Autodesk Fusion 360 part; units mm, degrees
(part 5 of 9)
  spline S340 degree 3 poles (68.6306, 8.3911) (68.6068, 8.8872) (68.4218, 9.22) (68.0776, 9.3884) knots 0 0 0 0 1 1 1 1
  spline S341 degree 3 poles (68.0776, 9.3884) (67.8813, 9.4814) (67.5733, 9.528) (67.1526, 9.528) knots 0 0 0 0 1 1 1 1
  line L476 (67.1526, 9.528) -> (64.8117, 9.528)
  line L477 (64.8117, 9.528) -> (64.8117, 6.2723)
  line L478 (64.8117, 6.2723) -> (63.7833, 6.2723)
  line L479 (63.7833, 6.2723) -> (63.7833, 13.8636)
  line L480 (81.4443, 13.8636) -> (81.4443, 9.1714)
  spline S342 degree 3 poles (81.4443, 9.1714) (81.4443, 8.6205) (81.5476, 8.1616) (81.7543, 7.7968) knots 0 0 0 0 1 1 1 1
  spline S343 degree 3 poles (81.7543, 7.7968) (82.0613, 7.2459) (82.5781, 6.97) (83.3046, 6.97) knots 0 0 0 0 1 1 1 1
  spline S344 degree 3 poles (83.3046, 6.97) (84.1759, 6.97) (84.7691, 7.2676) (85.0823, 7.864) knots 0 0 0 0 1 1 1 1
  spline S345 degree 3 poles (85.0823, 7.864) (85.2508, 8.1875) (85.3355, 8.6236) (85.3355, 9.1714) knots 0 0 0 0 1 1 1 1
  line L481 (85.3355, 9.1714) -> (85.3355, 13.8636)
  line L482 (85.3355, 13.8636) -> (86.3794, 13.8636)
  line L483 (86.3794, 13.8636) -> (86.3794, 9.6003)
  spline S346 degree 3 poles (86.3794, 9.6003) (86.3794, 8.667) (86.2533, 7.9487) (86.0021, 7.4454) knots 0 0 0 0 1 1 1 1
  spline S347 degree 3 poles (86.0021, 7.4454) (85.5401, 6.5287) (84.6689, 6.0708) (83.3873, 6.0708) knots 0 0 0 0 1 1 1 1
  spline S348 degree 3 poles (83.3873, 6.0708) (82.1057, 6.0708) (81.2355, 6.5287) (80.7776, 7.4454) knots 0 0 0 0 1 1 1 1
  spline S349 degree 3 poles (80.7776, 7.4454) (80.5265, 7.9487) (80.4004, 8.667) (80.4004, 9.6003) knots 0 0 0 0 1 1 1 1
  line L484 (80.4004, 9.6003) -> (80.4004, 13.8636)
  line L485 (80.4004, 13.8636) -> (81.4443, 13.8636)
  line L486 (83.8782, 15.6619) -> (84.8446, 15.6619)
  line L487 (84.8446, 15.6619) -> (84.8446, 14.5871)
  line L488 (84.8446, 14.5871) -> (83.8782, 14.5871)
  line L489 (83.8782, 14.5871) -> (83.8782, 15.6619)
  line L490 (82.1729, 15.6619) -> (83.1393, 15.6619)
  line L491 (83.1393, 15.6619) -> (83.1393, 14.5871)
  line L492 (83.1393, 14.5871) -> (82.1729, 14.5871)
  line L493 (82.1729, 14.5871) -> (82.1729, 15.6619)
  line L494 (-85.4675, -4.6366) -> (-83.2868, -11.1013)
  line L495 (-83.2868, -11.1013) -> (-81.1319, -4.6366)
  line L496 (-81.1319, -4.6366) -> (-79.9795, -4.6366)
  line L497 (-79.9795, -4.6366) -> (-82.7493, -12.2278)
  line L498 (-82.7493, -12.2278) -> (-83.8397, -12.2278)
  line L499 (-83.8397, -12.2278) -> (-86.6044, -4.6366)
  line L500 (-86.6044, -4.6366) -> (-85.4675, -4.6366)
  line L501 (-67.1058, -4.6366) -> (-66.0671, -4.6366)
  line L502 (-66.0671, -4.6366) -> (-66.0671, -12.2278)
  line L503 (-66.0671, -12.2278) -> (-67.1058, -12.2278)
  line L504 (-67.1058, -12.2278) -> (-67.1058, -4.6366)
  line L505 (-52.6313, -4.6366) -> (-47.0967, -4.6366)
  line L506 (-47.0967, -4.6366) -> (-47.0967, -5.5667)
  line L507 (-47.0967, -5.5667) -> (-51.6287, -5.5667)
  line L508 (-51.6287, -5.5667) -> (-51.6287, -7.8715)
  line L509 (-51.6287, -7.8715) -> (-47.4378, -7.8715)
  line L510 (-47.4378, -7.8715) -> (-47.4378, -8.75)
  line L511 (-47.4378, -8.75) -> (-51.6287, -8.75)
  line L512 (-51.6287, -8.75) -> (-51.6287, -11.3235)
  line L513 (-51.6287, -11.3235) -> (-47.0192, -11.3235)
  line L514 (-47.0192, -11.3235) -> (-47.0192, -12.2278)
  line L515 (-47.0192, -12.2278) -> (-52.6313, -12.2278)
  line L516 (-52.6313, -12.2278) -> (-52.6313, -4.6366)
  spline S350 degree 3 poles (-32.8237, -8.1144) (-32.341, -8.1144) (-31.9597, -8.0183) (-31.6796, -7.825) knots 0 0 0 0 1 1 1 1
  spline S351 degree 3 poles (-31.6796, -7.825) (-31.3985, -7.6317) (-31.2579, -7.2845) (-31.2579, -6.7811) knots 0 0 0 0 1 1 1 1
  spline S352 degree 3 poles (-31.2579, -6.7811) (-31.2579, -6.2406) (-31.4543, -5.8716) (-31.847, -5.6753) knots 0 0 0 0 1 1 1 1
  spline S353 degree 3 poles (-31.847, -5.6753) (-32.0568, -5.5719) (-32.3379, -5.5202) (-32.6893, -5.5202) knots 0 0 0 0 1 1 1 1
  line L517 (-32.6893, -5.5202) -> (-35.2008, -5.5202)
  line L518 (-35.2008, -5.5202) -> (-35.2008, -8.1144)
  line L519 (-35.2008, -8.1144) -> (-32.8237, -8.1144)
  line L520 (-36.2292, -4.6366) -> (-32.7152, -4.6366)
  spline S354 degree 3 poles (-32.7152, -4.6366) (-32.1364, -4.6366) (-31.6589, -4.7213) (-31.2837, -4.8898) knots 0 0 0 0 1 1 1 1
  spline S355 degree 3 poles (-31.2837, -4.8898) (-30.5706, -5.2133) (-30.214, -5.8117) (-30.214, -6.6829) knots 0 0 0 0 1 1 1 1
  spline S356 degree 3 poles (-30.214, -6.6829) (-30.214, -7.1377) (-30.3081, -7.5098) (-30.4951, -7.7992) knots 0 0 0 0 1 1 1 1
  spline S357 degree 3 poles (-30.4951, -7.7992) (-30.6833, -8.0885) (-30.9458, -8.3211) (-31.2837, -8.4968) knots 0 0 0 0 1 1 1 1
  spline S358 degree 3 poles (-31.2837, -8.4968) (-30.9871, -8.6177) (-30.7639, -8.7758) (-30.615, -8.9722) knots 0 0 0 0 1 1 1 1
  spline S359 degree 3 poles (-30.615, -8.9722) (-30.4652, -9.1686) (-30.3815, -9.4869) (-30.3639, -9.9282) knots 0 0 0 0 1 1 1 1
  line L521 (-30.3639, -9.9282) -> (-30.3277, -10.9462)
  spline S360 degree 3 poles (-30.3277, -10.9462) (-30.3174, -11.2356) (-30.2936, -11.4506) (-30.2554, -11.5922) knots 0 0 0 0 1 1 1 1
  spline S361 degree 3 poles (-30.2554, -11.5922) (-30.1934, -11.833) (-30.0828, -11.988) (-29.9246, -12.0573) knots 0 0 0 0 1 1 1 1
  line L522 (-29.9246, -12.0573) -> (-29.9246, -12.2278)
  line L523 (-29.9246, -12.2278) -> (-31.1855, -12.2278)
  spline S362 degree 3 poles (-31.1855, -12.2278) (-31.2197, -12.1627) (-31.2476, -12.078) (-31.2682, -11.9746) knots 0 0 0 0 1 1 1 1
  spline S363 degree 3 poles (-31.2682, -11.9746) (-31.2889, -11.8713) (-31.3065, -11.6718) (-31.3199, -11.3752) knots 0 0 0 0 1 1 1 1
  line L524 (-31.3199, -11.3752) -> (-31.3819, -10.1091)
  spline S364 degree 3 poles (-31.3819, -10.1091) (-31.4057, -9.613) (-31.5907, -9.2802) (-31.9349, -9.1117) knots 0 0 0 0 1 1 1 1
  spline S365 degree 3 poles (-31.9349, -9.1117) (-32.1312, -9.0187) (-32.4392, -8.9722) (-32.8599, -8.9722) knots 0 0 0 0 1 1 1 1
  line L525 (-32.8599, -8.9722) -> (-35.2008, -8.9722)
  line L526 (-35.2008, -8.9722) -> (-35.2008, -12.2278)
  line L527 (-35.2008, -12.2278) -> (-36.2292, -12.2278)
  line L528 (-36.2292, -12.2278) -> (-36.2292, -4.6366)
  line L529 (-17.0996, -4.6366) -> (-16.0609, -4.6366)
  line L530 (-16.0609, -4.6366) -> (-16.0609, -12.2278)
  line L531 (-16.0609, -12.2278) -> (-17.0996, -12.2278)
  line L532 (-17.0996, -12.2278) -> (-17.0996, -4.6366)
  line L533 (-2.3284, -4.6366) -> (2.9374, -4.6366)
  line L534 (2.9374, -4.6366) -> (2.9374, -5.5667)
  line L535 (2.9374, -5.5667) -> (-1.3, -5.5667)
  line L536 (-1.3, -5.5667) -> (-1.3, -7.8715)
  line L537 (-1.3, -7.8715) -> (2.4258, -7.8715)
  line L538 (2.4258, -7.8715) -> (2.4258, -8.7758)
  line L539 (2.4258, -8.7758) -> (-1.3, -8.7758)
  line L540 (-1.3, -8.7758) -> (-1.3, -12.2278)
  line L541 (-1.3, -12.2278) -> (-2.3284, -12.2278)
  line L542 (-2.3284, -12.2278) -> (-2.3284, -4.6366)
  line L543 (14.7693, -4.6366) -> (14.7693, -9.3288)
  spline S366 degree 3 poles (14.7693, -9.3288) (14.7693, -9.8796) (14.8726, -10.3385) (15.0793, -10.7034) knots 0 0 0 0 1 1 1 1
  spline S367 degree 3 poles (15.0793, -10.7034) (15.3863, -11.2542) (15.9031, -11.5302) (16.6296, -11.5302) knots 0 0 0 0 1 1 1 1
  spline S368 degree 3 poles (16.6296, -11.5302) (17.5009, -11.5302) (18.0941, -11.2325) (18.4073, -10.6362) knots 0 0 0 0 1 1 1 1
  spline S369 degree 3 poles (18.4073, -10.6362) (18.5758, -10.3127) (18.6605, -9.8765) (18.6605, -9.3288) knots 0 0 0 0 1 1 1 1
  line L544 (18.6605, -9.3288) -> (18.6605, -4.6366)
  line L545 (18.6605, -4.6366) -> (19.7044, -4.6366)
  line L546 (19.7044, -4.6366) -> (19.7044, -8.8999)
  spline S370 degree 3 poles (19.7044, -8.8999) (19.7044, -9.8331) (19.5783, -10.5514) (19.3271, -11.0548) knots 0 0 0 0 1 1 1 1
  spline S371 degree 3 poles (19.3271, -11.0548) (18.8651, -11.9715) (17.9939, -12.4294) (16.7123, -12.4294) knots 0 0 0 0 1 1 1 1
  spline S372 degree 3 poles (16.7123, -12.4294) (15.4307, -12.4294) (14.5605, -11.9715) (14.1026, -11.0548) knots 0 0 0 0 1 1 1 1
  spline S373 degree 3 poles (14.1026, -11.0548) (13.8515, -10.5514) (13.7254, -9.8331) (13.7254, -8.8999) knots 0 0 0 0 1 1 1 1
  line L547 (13.7254, -8.8999) -> (13.7254, -4.6366)
  line L548 (13.7254, -4.6366) -> (14.7693, -4.6366)
  line L549 (17.2032, -2.8382) -> (18.1696, -2.8382)
  line L550 (18.1696, -2.8382) -> (18.1696, -3.9131)
  line L551 (18.1696, -3.9131) -> (17.2032, -3.9131)
  line L552 (17.2032, -3.9131) -> (17.2032, -2.8382)
  line L553 (15.4979, -2.8382) -> (16.4643, -2.8382)
  line L554 (16.4643, -2.8382) -> (16.4643, -3.9131)
  line L555 (16.4643, -3.9131) -> (15.4979, -3.9131)
  line L556 (15.4979, -3.9131) -> (15.4979, -2.8382)
  line L557 (31.0091, -4.6366) -> (36.2749, -4.6366)
  line L558 (36.2749, -4.6366) -> (36.2749, -5.5667)
  line L559 (36.2749, -5.5667) -> (32.0375, -5.5667)
  line L560 (32.0375, -5.5667) -> (32.0375, -7.8715)
  line L561 (32.0375, -7.8715) -> (35.7633, -7.8715)
  line L562 (35.7633, -7.8715) -> (35.7633, -8.7758)
  line L563 (35.7633, -8.7758) -> (32.0375, -8.7758)
  line L564 (32.0375, -8.7758) -> (32.0375, -12.2278)
  line L565 (32.0375, -12.2278) -> (31.0091, -12.2278)
  line L566 (31.0091, -12.2278) -> (31.0091, -4.6366)
  line L567 (49.5754, -4.6366) -> (50.6141, -4.6366)
  line L568 (50.6141, -4.6366) -> (50.6141, -12.2278)
  line L569 (50.6141, -12.2278) -> (49.5754, -12.2278)
  line L570 (49.5754, -12.2278) -> (49.5754, -4.6366)
  spline S374 degree 3 poles (64.6236, -9.7784) (64.6474, -10.2093) (64.7497, -10.5587) (64.9285, -10.8274) knots 0 0 0 0 1 1 1 1
  spline S375 degree 3 poles (64.9285, -10.8274) (65.2695, -11.3307) (65.8711, -11.5819) (66.732, -11.5819) knots 0 0 0 0 1 1 1 1
  spline S376 degree 3 poles (66.732, -11.5819) (67.1175, -11.5819) (67.4689, -11.5271) (67.7862, -11.4165) knots 0 0 0 0 1 1 1 1
  spline S377 degree 3 poles (67.7862, -11.4165) (68.3991, -11.2026) (68.706, -10.8202) (68.706, -10.2693) knots 0 0 0 0 1 1 1 1
  spline S378 degree 3 poles (68.706, -10.2693) (68.706, -9.8559) (68.5768, -9.5613) (68.3185, -9.3856) knots 0 0 0 0 1 1 1 1
  spline S379 degree 3 poles (68.3185, -9.3856) (68.057, -9.213) (67.6467, -9.0632) (67.0886, -8.936) knots 0 0 0 0 1 1 1 1
  line L571 (67.0886, -8.936) -> (66.0602, -8.7035)
  spline S380 degree 3 poles (66.0602, -8.7035) (65.3884, -8.5516) (64.913, -8.3852) (64.6339, -8.2022) knots 0 0 0 0 1 1 1 1
  spline S381 degree 3 poles (64.6339, -8.2022) (64.1513, -7.8849) (63.9105, -7.4116) (63.9105, -6.7811) knots 0 0 0 0 1 1 1 1
  spline S382 degree 3 poles (63.9105, -6.7811) (63.9105, -6.099) (64.1461, -5.5388) (64.6184, -5.1016) knots 0 0 0 0 1 1 1 1
  spline S383 degree 3 poles (64.6184, -5.1016) (65.0907, -4.6645) (65.7584, -4.4454) (66.6235, -4.4454) knots 0 0 0 0 1 1 1 1
  spline S384 degree 3 poles (66.6235, -4.4454) (67.4193, -4.4454) (68.0952, -4.6376) (68.6523, -5.0221) knots 0 0 0 0 1 1 1 1
  spline S385 degree 3 poles (68.6523, -5.0221) (69.2083, -5.4055) (69.4863, -6.0194) (69.4863, -6.8638) knots 0 0 0 0 1 1 1 1
  line L572 (69.4863, -6.8638) -> (68.52, -6.8638)
  spline S386 degree 3 poles (68.52, -6.8638) (68.4683, -6.4576) (68.3577, -6.1455) (68.1893, -5.9285) knots 0 0 0 0 1 1 1 1
  spline S387 degree 3 poles (68.1893, -5.9285) (67.8761, -5.5326) (67.3438, -5.3342) (66.5925, -5.3342) knots 0 0 0 0 1 1 1 1
  spline S388 degree 3 poles (66.5925, -5.3342) (65.9858, -5.3342) (65.5507, -5.4613) (65.2851, -5.7166) knots 0 0 0 0 1 1 1 1
  spline S389 degree 3 poles (65.2851, -5.7166) (65.0194, -5.9719) (64.8871, -6.2675) (64.8871, -6.6054) knots 0 0 0 0 1 1 1 1
  spline S390 degree 3 poles (64.8871, -6.6054) (64.8871, -6.9775) (65.0422, -7.2493) (65.3522, -7.4219) knots 0 0 0 0 1 1 1 1
  spline S391 degree 3 poles (65.3522, -7.4219) (65.5558, -7.5325) (66.0158, -7.67) (66.732, -7.8353) knots 0 0 0 0 1 1 1 1
  line L573 (66.732, -7.8353) -> (67.7965, -8.0782)
  spline S392 degree 3 poles (67.7965, -8.0782) (68.3102, -8.195) (68.706, -8.3552) (68.9851, -8.5588) knots 0 0 0 0 1 1 1 1
  spline S393 degree 3 poles (68.9851, -8.5588) (69.4677, -8.9133) (69.7086, -9.429) (69.7086, -10.1039) knots 0 0 0 0 1 1 1 1
  spline S394 degree 3 poles (69.7086, -10.1039) (69.7086, -10.9442) (69.4026, -11.5457) (68.7908, -11.9074) knots 0 0 0 0 1 1 1 1
  spline S395 degree 3 poles (68.7908, -11.9074) (68.18, -12.2692) (67.4689, -12.45) (66.6596, -12.45) knots 0 0 0 0 1 1 1 1
  spline S396 degree 3 poles (66.6596, -12.45) (65.716, -12.45) (64.9771, -12.2092) (64.4427, -11.7266) knots 0 0 0 0 1 1 1 1
  spline S397 degree 3 poles (64.4427, -11.7266) (63.9084, -11.248) (63.6469, -10.5979) (63.6572, -9.7784) knots 0 0 0 0 1 1 1 1
  line L574 (63.6572, -9.7784) -> (64.6236, -9.7784)
  line L575 (86.4414, -4.6366) -> (86.4414, -5.5409)
  line L576 (86.4414, -5.5409) -> (83.8834, -5.5409)
  line L577 (83.8834, -5.5409) -> (83.8834, -12.2278)
  line L578 (83.8834, -12.2278) -> (82.8395, -12.2278)
  line L579 (82.8395, -12.2278) -> (82.8395, -5.5409)
  line L580 (82.8395, -5.5409) -> (80.2816, -5.5409)
  line L581 (80.2816, -5.5409) -> (80.2816, -4.6366)
  line L582 (80.2816, -4.6366) -> (86.4414, -4.6366)
  spline S398 degree 3 poles (-85.3952, -28.2785) (-85.3714, -28.7095) (-85.2691, -29.0588) (-85.0903, -29.3276) knots 0 0 0 0 1 1 1 1
  spline S399 degree 3 poles (-85.0903, -29.3276) (-84.7492, -29.8309) (-84.1477, -30.082) (-83.2868, -30.082) knots 0 0 0 0 1 1 1 1
  spline S400 degree 3 poles (-83.2868, -30.082) (-82.9013, -30.082) (-82.5499, -30.0273) (-82.2326, -29.9167) knots 0 0 0 0 1 1 1 1
  spline S401 degree 3 poles (-82.2326, -29.9167) (-81.6197, -29.7027) (-81.3127, -29.3203) (-81.3127, -28.7694) knots 0 0 0 0 1 1 1 1
  spline S402 degree 3 poles (-81.3127, -28.7694) (-81.3127, -28.356) (-81.4419, -28.0615) (-81.7003, -27.8858) knots 0 0 0 0 1 1 1 1
  spline S403 degree 3 poles (-81.7003, -27.8858) (-81.9618, -27.7132) (-82.3721, -27.5633) (-82.9302, -27.4362) knots 0 0 0 0 1 1 1 1
  line L583 (-82.9302, -27.4362) -> (-83.9586, -27.2037)
  spline S404 degree 3 poles (-83.9586, -27.2037) (-84.6303, -27.0517) (-85.1058, -26.8853) (-85.3848, -26.7024) knots 0 0 0 0 1 1 1 1
  spline S405 degree 3 poles (-85.3848, -26.7024) (-85.8675, -26.3851) (-86.1083, -25.9117) (-86.1083, -25.2813) knots 0 0 0 0 1 1 1 1
  spline S406 degree 3 poles (-86.1083, -25.2813) (-86.1083, -24.5992) (-85.8726, -24.039) (-85.4003, -23.6018) knots 0 0 0 0 1 1 1 1
  spline S407 degree 3 poles (-85.4003, -23.6018) (-84.928, -23.1646) (-84.2603, -22.9455) (-83.3953, -22.9455) knots 0 0 0 0 1 1 1 1
  spline S408 degree 3 poles (-83.3953, -22.9455) (-82.5995, -22.9455) (-81.9235, -23.1378) (-81.3665, -23.5222) knots 0 0 0 0 1 1 1 1
  spline S409 degree 3 poles (-81.3665, -23.5222) (-80.8104, -23.9057) (-80.5324, -24.5196) (-80.5324, -25.364) knots 0 0 0 0 1 1 1 1
  line L584 (-80.5324, -25.364) -> (-81.4988, -25.364)
  spline S410 degree 3 poles (-81.4988, -25.364) (-81.5504, -24.9578) (-81.661, -24.6457) (-81.8295, -24.4286) knots 0 0 0 0 1 1 1 1
  spline S411 degree 3 poles (-81.8295, -24.4286) (-82.1426, -24.0328) (-82.6749, -23.8344) (-83.4263, -23.8344) knots 0 0 0 0 1 1 1 1
  spline S412 degree 3 poles (-83.4263, -23.8344) (-84.033, -23.8344) (-84.4681, -23.9615) (-84.7337, -24.2168) knots 0 0 0 0 1 1 1 1
  spline S413 degree 3 poles (-84.7337, -24.2168) (-84.9993, -24.472) (-85.1316, -24.7676) (-85.1316, -25.1056) knots 0 0 0 0 1 1 1 1
  spline S414 degree 3 poles (-85.1316, -25.1056) (-85.1316, -25.4777) (-84.9766, -25.7495) (-84.6665, -25.9221) knots 0 0 0 0 1 1 1 1
  spline S415 degree 3 poles (-84.6665, -25.9221) (-84.4629, -26.0327) (-84.003, -26.1701) (-83.2868, -26.3355) knots 0 0 0 0 1 1 1 1
  line L585 (-83.2868, -26.3355) -> (-82.2222, -26.5784)
  spline S416 degree 3 poles (-82.2222, -26.5784) (-81.7086, -26.6952) (-81.3127, -26.8554) (-81.0337, -27.059) knots 0 0 0 0 1 1 1 1
  spline S417 degree 3 poles (-81.0337, -27.059) (-80.551, -27.4135) (-80.3102, -27.9292) (-80.3102, -28.6041) knots 0 0 0 0 1 1 1 1
  spline S418 degree 3 poles (-80.3102, -28.6041) (-80.3102, -29.4443) (-80.6161, -30.0459) (-81.228, -30.4076) knots 0 0 0 0 1 1 1 1
  spline S419 degree 3 poles (-81.228, -30.4076) (-81.8388, -30.7693) (-82.5499, -30.9502) (-83.3591, -30.9502) knots 0 0 0 0 1 1 1 1
  spline S420 degree 3 poles (-83.3591, -30.9502) (-84.3027, -30.9502) (-85.0417, -30.7094) (-85.576, -30.2267) knots 0 0 0 0 1 1 1 1
  spline S421 degree 3 poles (-85.576, -30.2267) (-86.1104, -29.7482) (-86.3718, -29.0981) (-86.3615, -28.2785) knots 0 0 0 0 1 1 1 1
  line L586 (-86.3615, -28.2785) -> (-85.3952, -28.2785)
  line L587 (-65.5018, -27.6171) -> (-66.6542, -24.2633)
  line L588 (-66.6542, -24.2633) -> (-67.8789, -27.6171)
  line L589 (-67.8789, -27.6171) -> (-65.5018, -27.6171)
  line L590 (-67.1916, -23.1367) -> (-66.0289, -23.1367)
  line L591 (-66.0289, -23.1367) -> (-63.2745, -30.728)
  line L592 (-63.2745, -30.728) -> (-64.4011, -30.728)
  line L593 (-64.4011, -30.728) -> (-65.1711, -28.4542)
  line L594 (-65.1711, -28.4542) -> (-68.1735, -28.4542)
  line L595 (-68.1735, -28.4542) -> (-68.9951, -30.728)
  line L596 (-68.9951, -30.728) -> (-70.0493, -30.728)
  line L597 (-70.0493, -30.728) -> (-67.1916, -23.1367)
  line L598 (-66.2924, -21.3384) -> (-65.3261, -21.3384)
  line L599 (-65.3261, -21.3384) -> (-65.3261, -22.4132)
  line L600 (-65.3261, -22.4132) -> (-66.2924, -22.4132)
  line L601 (-66.2924, -22.4132) -> (-66.2924, -21.3384)
  line L602 (-67.9978, -21.3384) -> (-67.0314, -21.3384)
  line L603 (-67.0314, -21.3384) -> (-67.0314, -22.4132)
  line L604 (-67.0314, -22.4132) -> (-67.9978, -22.4132)
  line L605 (-67.9978, -22.4132) -> (-67.9978, -21.3384)
  spline S422 degree 3 poles (-49.8232, -22.93) (-48.862, -22.93) (-48.1158, -23.1832) (-47.5856, -23.6897) knots 0 0 0 0 1 1 1 1
  spline S423 degree 3 poles (-47.5856, -23.6897) (-47.0554, -24.1961) (-46.7608, -24.7718) (-46.7019, -25.4156) knots 0 0 0 0 1 1 1 1
  line L606 (-46.7019, -25.4156) -> (-47.7044, -25.4156)
  spline S424 degree 3 poles (-47.7044, -25.4156) (-47.8181, -24.9268) (-48.0445, -24.5392) (-48.3835, -24.2529) knots 0 0 0 0 1 1 1 1
  spline S425 degree 3 poles (-48.3835, -24.2529) (-48.7235, -23.9666) (-49.2, -23.824) (-49.8128, -23.824) knots 0 0 0 0 1 1 1 1
  spline S426 degree 3 poles (-49.8128, -23.824) (-50.5601, -23.824) (-51.1637, -24.0865) (-51.6246, -24.6116) knots 0 0 0 0 1 1 1 1
  spline S427 degree 3 poles (-51.6246, -24.6116) (-52.0845, -25.1376) (-52.314, -25.9427) (-52.314, -27.028) knots 0 0 0 0 1 1 1 1
  spline S428 degree 3 poles (-52.314, -27.028) (-52.314, -27.9168) (-52.1062, -28.6382) (-51.6908, -29.1901) knots 0 0 0 0 1 1 1 1
  spline S429 degree 3 poles (-51.6908, -29.1901) (-51.2763, -29.743) (-50.6572, -30.02) (-49.8335, -30.02) knots 0 0 0 0 1 1 1 1
  spline S430 degree 3 poles (-49.8335, -30.02) (-49.0759, -30.02) (-48.4982, -29.7286) (-48.1023, -29.1467) knots 0 0 0 0 1 1 1 1
  spline S431 degree 3 poles (-48.1023, -29.1467) (-47.8925, -28.8397) (-47.7354, -28.4367) (-47.6321, -27.9375) knots 0 0 0 0 1 1 1 1
  line L607 (-47.6321, -27.9375) -> (-46.6296, -27.9375)
  spline S432 degree 3 poles (-46.6296, -27.9375) (-46.7195, -28.7364) (-47.0151, -29.4071) (-47.5184, -29.9477) knots 0 0 0 0 1 1 1 1
  spline S433 degree 3 poles (-47.5184, -29.9477) (-48.1209, -30.5988) (-48.9343, -30.9244) (-49.9575, -30.9244) knots 0 0 0 0 1 1 1 1
  spline S434 degree 3 poles (-49.9575, -30.9244) (-50.8391, -30.9244) (-51.5802, -30.6577) (-52.1796, -30.1234) knots 0 0 0 0 1 1 1 1
  spline S435 degree 3 poles (-52.1796, -30.1234) (-52.9682, -29.4175) (-53.363, -28.3271) (-53.363, -26.8523) knots 0 0 0 0 1 1 1 1
  spline S436 degree 3 poles (-53.363, -26.8523) (-53.363, -25.7329) (-53.0664, -24.8141) (-52.4742, -24.0979) knots 0 0 0 0 1 1 1 1
  spline S437 degree 3 poles (-52.4742, -24.0979) (-51.8334, -23.3197) (-50.9497, -22.93) (-49.8232, -22.93) knots 0 0 0 0 1 1 1 1
  line L608 (-36.3274, -23.1367) -> (-35.2887, -23.1367)
  line L609 (-35.2887, -23.1367) -> (-35.2887, -26.2735)
  line L610 (-35.2887, -26.2735) -> (-31.3406, -26.2735)
  line L611 (-31.3406, -26.2735) -> (-31.3406, -23.1367)
  line L612 (-31.3406, -23.1367) -> (-30.3019, -23.1367)
  line L613 (-30.3019, -23.1367) -> (-30.3019, -30.728)
  line L614 (-30.3019, -30.728) -> (-31.3406, -30.728)
  line L615 (-31.3406, -30.728) -> (-31.3406, -27.1778)
  line L616 (-31.3406, -27.1778) -> (-35.2887, -27.1778)
  line L617 (-35.2887, -27.1778) -> (-35.2887, -30.728)
  line L618 (-35.2887, -30.728) -> (-36.3274, -30.728)
  line L619 (-36.3274, -30.728) -> (-36.3274, -23.1367)
  spline S438 degree 3 poles (-18.7202, -28.2785) (-18.6964, -28.7095) (-18.5941, -29.0588) (-18.4153, -29.3276) knots 0 0 0 0 1 1 1 1
  spline S439 degree 3 poles (-18.4153, -29.3276) (-18.0742, -29.8309) (-17.4727, -30.082) (-16.6118, -30.082) knots 0 0 0 0 1 1 1 1
  spline S440 degree 3 poles (-16.6118, -30.082) (-16.2263, -30.082) (-15.8749, -30.0273) (-15.5576, -29.9167) knots 0 0 0 0 1 1 1 1
  spline S441 degree 3 poles (-15.5576, -29.9167) (-14.9447, -29.7027) (-14.6377, -29.3203) (-14.6377, -28.7694) knots 0 0 0 0 1 1 1 1
  spline S442 degree 3 poles (-14.6377, -28.7694) (-14.6377, -28.356) (-14.7669, -28.0615) (-15.0253, -27.8858) knots 0 0 0 0 1 1 1 1
  spline S443 degree 3 poles (-15.0253, -27.8858) (-15.2868, -27.7132) (-15.6971, -27.5633) (-16.2552, -27.4362) knots 0 0 0 0 1 1 1 1
  line L620 (-16.2552, -27.4362) -> (-17.2836, -27.2037)
  spline S444 degree 3 poles (-17.2836, -27.2037) (-17.9553, -27.0517) (-18.4308, -26.8853) (-18.7098, -26.7024) knots 0 0 0 0 1 1 1 1
  spline S445 degree 3 poles (-18.7098, -26.7024) (-19.1925, -26.3851) (-19.4333, -25.9117) (-19.4333, -25.2813) knots 0 0 0 0 1 1 1 1
  spline S446 degree 3 poles (-19.4333, -25.2813) (-19.4333, -24.5992) (-19.1976, -24.039) (-18.7253, -23.6018) knots 0 0 0 0 1 1 1 1
  spline S447 degree 3 poles (-18.7253, -23.6018) (-18.253, -23.1646) (-17.5853, -22.9455) (-16.7203, -22.9455) knots 0 0 0 0 1 1 1 1
  spline S448 degree 3 poles (-16.7203, -22.9455) (-15.9245, -22.9455) (-15.2485, -23.1378) (-14.6915, -23.5222) knots 0 0 0 0 1 1 1 1
  spline S449 degree 3 poles (-14.6915, -23.5222) (-14.1354, -23.9057) (-13.8574, -24.5196) (-13.8574, -25.364) knots 0 0 0 0 1 1 1 1
  line L621 (-13.8574, -25.364) -> (-14.8238, -25.364)
  spline S450 degree 3 poles (-14.8238, -25.364) (-14.8754, -24.9578) (-14.986, -24.6457) (-15.1545, -24.4286) knots 0 0 0 0 1 1 1 1
  spline S451 degree 3 poles (-15.1545, -24.4286) (-15.4676, -24.0328) (-15.9999, -23.8344) (-16.7513, -23.8344) knots 0 0 0 0 1 1 1 1
  spline S452 degree 3 poles (-16.7513, -23.8344) (-17.358, -23.8344) (-17.7931, -23.9615) (-18.0587, -24.2168) knots 0 0 0 0 1 1 1 1
  spline S453 degree 3 poles (-18.0587, -24.2168) (-18.3243, -24.472) (-18.4566, -24.7676) (-18.4566, -25.1056) knots 0 0 0 0 1 1 1 1
  spline S454 degree 3 poles (-18.4566, -25.1056) (-18.4566, -25.4777) (-18.3016, -25.7495) (-17.9915, -25.9221) knots 0 0 0 0 1 1 1 1
  spline S455 degree 3 poles (-17.9915, -25.9221) (-17.7879, -26.0327) (-17.328, -26.1701) (-16.6118, -26.3355) knots 0 0 0 0 1 1 1 1
  line L622 (-16.6118, -26.3355) -> (-15.5472, -26.5784)
  spline S456 degree 3 poles (-15.5472, -26.5784) (-15.0336, -26.6952) (-14.6377, -26.8554) (-14.3587, -27.059) knots 0 0 0 0 1 1 1 1
  spline S457 degree 3 poles (-14.3587, -27.059) (-13.876, -27.4135) (-13.6352, -27.9292) (-13.6352, -28.6041) knots 0 0 0 0 1 1 1 1
  spline S458 degree 3 poles (-13.6352, -28.6041) (-13.6352, -29.4443) (-13.9411, -30.0459) (-14.553, -30.4076) knots 0 0 0 0 1 1 1 1
  spline S459 degree 3 poles (-14.553, -30.4076) (-15.1638, -30.7693) (-15.8749, -30.9502) (-16.6841, -30.9502) knots 0 0 0 0 1 1 1 1
  spline S460 degree 3 poles (-16.6841, -30.9502) (-17.6277, -30.9502) (-18.3667, -30.7094) (-18.901, -30.2267) knots 0 0 0 0 1 1 1 1
  spline S461 degree 3 poles (-18.901, -30.2267) (-19.4354, -29.7482) (-19.6968, -29.0981) (-19.6865, -28.2785) knots 0 0 0 0 1 1 1 1
  line L623 (-19.6865, -28.2785) -> (-18.7202, -28.2785)
  line L624 (-0.4308, -23.1367) -> (0.6079, -23.1367)
  line L625 (0.6079, -23.1367) -> (0.6079, -30.728)
  line L626 (0.6079, -30.728) -> (-0.4308, -30.728)
  line L627 (-0.4308, -30.728) -> (-0.4308, -23.1367)
  spline S462 degree 3 poles (14.6173, -28.2785) (14.6411, -28.7095) (14.7434, -29.0588) (14.9222, -29.3276) knots 0 0 0 0 1 1 1 1
  spline S463 degree 3 poles (14.9222, -29.3276) (15.2633, -29.8309) (15.8648, -30.082) (16.7257, -30.082) knots 0 0 0 0 1 1 1 1
  spline S464 degree 3 poles (16.7257, -30.082) (17.1112, -30.082) (17.4626, -30.0273) (17.7799, -29.9167) knots 0 0 0 0 1 1 1 1
  spline S465 degree 3 poles (17.7799, -29.9167) (18.3928, -29.7027) (18.6998, -29.3203) (18.6998, -28.7694) knots 0 0 0 0 1 1 1 1
  spline S466 degree 3 poles (18.6998, -28.7694) (18.6998, -28.356) (18.5706, -28.0615) (18.3122, -27.8858) knots 0 0 0 0 1 1 1 1
  spline S467 degree 3 poles (18.3122, -27.8858) (18.0507, -27.7132) (17.6404, -27.5633) (17.0823, -27.4362) knots 0 0 0 0 1 1 1 1
  line L628 (17.0823, -27.4362) -> (16.0539, -27.2037)
  spline S468 degree 3 poles (16.0539, -27.2037) (15.3822, -27.0517) (14.9067, -26.8853) (14.6277, -26.7024) knots 0 0 0 0 1 1 1 1
  spline S469 degree 3 poles (14.6277, -26.7024) (14.145, -26.3851) (13.9042, -25.9117) (13.9042, -25.2813) knots 0 0 0 0 1 1 1 1
  spline S470 degree 3 poles (13.9042, -25.2813) (13.9042, -24.5992) (14.1399, -24.039) (14.6122, -23.6018) knots 0 0 0 0 1 1 1 1
  spline S471 degree 3 poles (14.6122, -23.6018) (15.0845, -23.1646) (15.7522, -22.9455) (16.6172, -22.9455) knots 0 0 0 0 1 1 1 1
  spline S472 degree 3 poles (16.6172, -22.9455) (17.413, -22.9455) (18.089, -23.1378) (18.646, -23.5222) knots 0 0 0 0 1 1 1 1
  spline S473 degree 3 poles (18.646, -23.5222) (19.2021, -23.9057) (19.4801, -24.5196) (19.4801, -25.364) knots 0 0 0 0 1 1 1 1
  line L629 (19.4801, -25.364) -> (18.5137, -25.364)
  spline S474 degree 3 poles (18.5137, -25.364) (18.4621, -24.9578) (18.3515, -24.6457) (18.183, -24.4286) knots 0 0 0 0 1 1 1 1
  spline S475 degree 3 poles (18.183, -24.4286) (17.8699, -24.0328) (17.3376, -23.8344) (16.5862, -23.8344) knots 0 0 0 0 1 1 1 1
  spline S476 degree 3 poles (16.5862, -23.8344) (15.9795, -23.8344) (15.5444, -23.9615) (15.2788, -24.2168) knots 0 0 0 0 1 1 1 1
  spline S477 degree 3 poles (15.2788, -24.2168) (15.0132, -24.472) (14.8809, -24.7676) (14.8809, -25.1056) knots 0 0 0 0 1 1 1 1
  spline S478 degree 3 poles (14.8809, -25.1056) (14.8809, -25.4777) (15.0359, -25.7495) (15.346, -25.9221) knots 0 0 0 0 1 1 1 1
  spline S479 degree 3 poles (15.346, -25.9221) (15.5496, -26.0327) (16.0095, -26.1701) (16.7257, -26.3355) knots 0 0 0 0 1 1 1 1
  line L630 (16.7257, -26.3355) -> (17.7903, -26.5784)
  spline S480 degree 3 poles (17.7903, -26.5784) (18.3039, -26.6952) (18.6998, -26.8554) (18.9788, -27.059) knots 0 0 0 0 1 1 1 1
  spline S481 degree 3 poles (18.9788, -27.059) (19.4615, -27.4135) (19.7023, -27.9292) (19.7023, -28.6041) knots 0 0 0 0 1 1 1 1
  spline S482 degree 3 poles (19.7023, -28.6041) (19.7023, -29.4443) (19.3964, -30.0459) (18.7845, -30.4076) knots 0 0 0 0 1 1 1 1
  spline S483 degree 3 poles (18.7845, -30.4076) (18.1737, -30.7693) (17.4626, -30.9502) (16.6534, -30.9502) knots 0 0 0 0 1 1 1 1
  spline S484 degree 3 poles (16.6534, -30.9502) (15.7098, -30.9502) (14.9708, -30.7094) (14.4365, -30.2267) knots 0 0 0 0 1 1 1 1
  spline S485 degree 3 poles (14.4365, -30.2267) (13.9021, -29.7482) (13.6407, -29.0981) (13.651, -28.2785) knots 0 0 0 0 1 1 1 1
  line L631 (13.651, -28.2785) -> (14.6173, -28.2785)
  line L632 (32.9067, -23.1367) -> (33.9454, -23.1367)
  line L633 (33.9454, -23.1367) -> (33.9454, -30.728)
  line L634 (33.9454, -30.728) -> (32.9067, -30.728)
  line L635 (32.9067, -30.728) -> (32.9067, -23.1367)
  spline S486 degree 3 poles (50.1356, -26.3458) (50.5697, -26.3458) (50.9076, -26.2859) (51.1484, -26.165) knots 0 0 0 0 1 1 1 1
  spline S487 degree 3 poles (51.1484, -26.165) (51.5278, -25.9758) (51.7169, -25.6348) (51.7169, -25.1418) knots 0 0 0 0 1 1 1 1
  spline S488 degree 3 poles (51.7169, -25.1418) (51.7169, -24.6457) (51.5153, -24.3118) (51.1123, -24.1392) knots 0 0 0 0 1 1 1 1
  spline S489 degree 3 poles (51.1123, -24.1392) (50.8849, -24.0431) (50.5469, -23.9945) (50.0994, -23.9945) knots 0 0 0 0 1 1 1 1
  line L636 (50.0994, -23.9945) -> (48.2649, -23.9945)
  line L637 (48.2649, -23.9945) -> (48.2649, -26.3458)
  line L638 (48.2649, -26.3458) -> (50.1356, -26.3458)
  spline S490 degree 3 poles (50.4818, -29.8495) (51.1123, -29.8495) (51.5619, -29.6666) (51.8306, -29.3017) knots 0 0 0 0 1 1 1 1
  spline S491 degree 3 poles (51.8306, -29.3017) (51.999, -29.0712) (52.0838, -28.7922) (52.0838, -28.4646) knots 0 0 0 0 1 1 1 1
  spline S492 degree 3 poles (52.0838, -28.4646) (52.0838, -27.9137) (51.8378, -27.5375) (51.3448, -27.338) knots 0 0 0 0 1 1 1 1
  spline S493 degree 3 poles (51.3448, -27.338) (51.0833, -27.2316) (50.7371, -27.1778) (50.3061, -27.1778) knots 0 0 0 0 1 1 1 1
  line L639 (50.3061, -27.1778) -> (48.2649, -27.1778)
  line L640 (48.2649, -27.1778) -> (48.2649, -29.8495)
  line L641 (48.2649, -29.8495) -> (50.4818, -29.8495)
  line L642 (47.2572, -23.1367) -> (50.518, -23.1367)
  spline S494 degree 3 poles (50.518, -23.1367) (51.4068, -23.1367) (52.0393, -23.4023) (52.4145, -23.9325) knots 0 0 0 0 1 1 1 1
  spline S495 degree 3 poles (52.4145, -23.9325) (52.6347, -24.2457) (52.7452, -24.6074) (52.7452, -25.0177) knots 0 0 0 0 1 1 1 1
  spline S496 degree 3 poles (52.7452, -25.0177) (52.7452, -25.4963) (52.6088, -25.889) (52.337, -26.196) knots 0 0 0 0 1 1 1 1
  spline S497 degree 3 poles (52.337, -26.196) (52.1954, -26.3582) (51.9928, -26.506) (51.7272, -26.6404) knots 0 0 0 0 1 1 1 1
  spline S498 degree 3 poles (51.7272, -26.6404) (52.1169, -26.7882) (52.4073, -26.9556) (52.6006, -27.1416) knots 0 0 0 0 1 1 1 1
  spline S499 degree 3 poles (52.6006, -27.1416) (52.9416, -27.4724) (53.1122, -27.9292) (53.1122, -28.5111) knots 0 0 0 0 1 1 1 1
  spline S500 degree 3 poles (53.1122, -28.5111) (53.1122, -28.9999) (52.9592, -29.4433) (52.6522, -29.8392) knots 0 0 0 0 1 1 1 1
  spline S501 degree 3 poles (52.6522, -29.8392) (52.1944, -30.4314) (51.4657, -30.728) (50.4663, -30.728) knots 0 0 0 0 1 1 1 1
  line L643 (50.4663, -30.728) -> (47.2572, -30.728)
  line L644 (47.2572, -30.728) -> (47.2572, -23.1367)
  line L645 (63.6593, -23.1367) -> (64.8737, -23.1367)
  line L646 (64.8737, -23.1367) -> (68.7081, -29.2862)
  line L647 (68.7081, -29.2862) -> (68.7081, -23.1367)
  line L648 (68.7081, -23.1367) -> (69.6848, -23.1367)
  line L649 (69.6848, -23.1367) -> (69.6848, -30.728)
  line L650 (69.6848, -30.728) -> (68.5324, -30.728)
  line L651 (68.5324, -30.728) -> (64.6412, -24.5837)
  line L652 (64.6412, -24.5837) -> (64.6412, -30.728)
  line L653 (64.6412, -30.728) -> (63.6593, -30.728)
  line L654 (63.6593, -30.728) -> (63.6593, -23.1367)
  line L655 (82.9129, -23.1367) -> (83.9516, -23.1367)
  line L656 (83.9516, -23.1367) -> (83.9516, -30.728)
  line L657 (83.9516, -30.728) -> (82.9129, -30.728)
  line L658 (82.9129, -30.728) -> (82.9129, -23.1367)
  line L659 (-82.1705, -46.1162) -> (-83.3229, -42.7624)
  line L660 (-83.3229, -42.7624) -> (-84.5477, -46.1162)
  line L661 (-84.5477, -46.1162) -> (-82.1705, -46.1162)
  line L662 (-83.8604, -41.6358) -> (-82.6976, -41.6358)
  line L663 (-82.6976, -41.6358) -> (-79.9433, -49.2271)
  line L664 (-79.9433, -49.2271) -> (-81.0698, -49.2271)
  line L665 (-81.0698, -49.2271) -> (-81.8398, -46.9534)
  line L666 (-81.8398, -46.9534) -> (-84.8422, -46.9534)
  line L667 (-84.8422, -46.9534) -> (-85.6639, -49.2271)
  line L668 (-85.6639, -49.2271) -> (-86.7181, -49.2271)
  line L669 (-86.7181, -49.2271) -> (-83.8604, -41.6358)
  spline S502 degree 3 poles (-66.4919, -41.4291) (-65.5307, -41.4291) (-64.7845, -41.6824) (-64.2543, -42.1888) knots 0 0 0 0 1 1 1 1
  spline S503 degree 3 poles (-64.2543, -42.1888) (-63.7241, -42.6952) (-63.4296, -43.2709) (-63.3707, -43.9148) knots 0 0 0 0 1 1 1 1
  line L670 (-63.3707, -43.9148) -> (-64.3732, -43.9148)
  spline S504 degree 3 poles (-64.3732, -43.9148) (-64.4869, -43.4259) (-64.7132, -43.0383) (-65.0522, -42.7521) knots 0 0 0 0 1 1 1 1
  spline S505 degree 3 poles (-65.0522, -42.7521) (-65.3922, -42.4658) (-65.8687, -42.3231) (-66.4816, -42.3231) knots 0 0 0 0 1 1 1 1
  spline S506 degree 3 poles (-66.4816, -42.3231) (-67.2288, -42.3231) (-67.8324, -42.5857) (-68.2934, -43.1107) knots 0 0 0 0 1 1 1 1
  spline S507 degree 3 poles (-68.2934, -43.1107) (-68.7533, -43.6368) (-68.9827, -44.4419) (-68.9827, -45.5271) knots 0 0 0 0 1 1 1 1
  spline S508 degree 3 poles (-68.9827, -45.5271) (-68.9827, -46.4159) (-68.775, -47.1373) (-68.3595, -47.6892) knots 0 0 0 0 1 1 1 1
  spline S509 degree 3 poles (-68.3595, -47.6892) (-67.9451, -48.2422) (-67.326, -48.5191) (-66.5023, -48.5191) knots 0 0 0 0 1 1 1 1
  spline S510 degree 3 poles (-66.5023, -48.5191) (-65.7447, -48.5191) (-65.1669, -48.2277) (-64.7711, -47.6458) knots 0 0 0 0 1 1 1 1
  spline S511 degree 3 poles (-64.7711, -47.6458) (-64.5613, -47.3389) (-64.4042, -46.9358) (-64.3008, -46.4366) knots 0 0 0 0 1 1 1 1
  line L671 (-64.3008, -46.4366) -> (-63.2983, -46.4366)
  spline S512 degree 3 poles (-63.2983, -46.4366) (-63.3882, -47.2355) (-63.6838, -47.9063) (-64.1872, -48.4468) knots 0 0 0 0 1 1 1 1
  spline S513 degree 3 poles (-64.1872, -48.4468) (-64.7897, -49.0979) (-65.6031, -49.4235) (-66.6263, -49.4235) knots 0 0 0 0 1 1 1 1
  spline S514 degree 3 poles (-66.6263, -49.4235) (-67.5079, -49.4235) (-68.2489, -49.1568) (-68.8484, -48.6225) knots 0 0 0 0 1 1 1 1
  spline S515 degree 3 poles (-68.8484, -48.6225) (-69.6369, -47.9166) (-70.0318, -46.8262) (-70.0318, -45.3514) knots 0 0 0 0 1 1 1 1
  spline S516 degree 3 poles (-70.0318, -45.3514) (-70.0318, -44.2321) (-69.7351, -43.3133) (-69.1429, -42.597) knots 0 0 0 0 1 1 1 1
  spline S517 degree 3 poles (-69.1429, -42.597) (-68.5021, -41.8188) (-67.6185, -41.4291) (-66.4919, -41.4291) knots 0 0 0 0 1 1 1 1
  line L672 (-52.9961, -41.6358) -> (-51.9574, -41.6358)
  line L673 (-51.9574, -41.6358) -> (-51.9574, -44.7726)
  line L674 (-51.9574, -44.7726) -> (-48.0093, -44.7726)
  line L675 (-48.0093, -44.7726) -> (-48.0093, -41.6358)
  line L676 (-48.0093, -41.6358) -> (-46.9706, -41.6358)
  line L677 (-46.9706, -41.6358) -> (-46.9706, -49.2271)
  line L678 (-46.9706, -49.2271) -> (-48.0093, -49.2271)
  line L679 (-48.0093, -49.2271) -> (-48.0093, -45.6769)
  line L680 (-48.0093, -45.6769) -> (-51.9574, -45.6769)
  line L681 (-51.9574, -45.6769) -> (-51.9574, -49.2271)
  line L682 (-51.9574, -49.2271) -> (-52.9961, -49.2271)
  line L683 (-52.9961, -49.2271) -> (-52.9961, -41.6358)
  line L684 (-30.2399, -41.6358) -> (-30.2399, -42.5402)
  line L685 (-30.2399, -42.5402) -> (-32.7979, -42.5402)
  line L686 (-32.7979, -42.5402) -> (-32.7979, -49.2271)
  line L687 (-32.7979, -49.2271) -> (-33.8417, -49.2271)
  line L688 (-33.8417, -49.2271) -> (-33.8417, -42.5402)
  line L689 (-33.8417, -42.5402) -> (-36.3997, -42.5402)
  line L690 (-36.3997, -42.5402) -> (-36.3997, -41.6358)
  line L691 (-36.3997, -41.6358) -> (-30.2399, -41.6358)
  line L692 (-17.0996, -41.6358) -> (-16.0609, -41.6358)
  line L693 (-16.0609, -41.6358) -> (-16.0609, -49.2271)
  line L694 (-16.0609, -49.2271) -> (-17.0996, -49.2271)
  line L695 (-17.0996, -49.2271) -> (-17.0996, -41.6358)
  line L696 (-3.0157, -41.6358) -> (-1.8013, -41.6358)
  line L697 (-1.8013, -41.6358) -> (2.0331, -47.7853)
  line L698 (2.0331, -47.7853) -> (2.0331, -41.6358)
  line L699 (2.0331, -41.6358) -> (3.0098, -41.6358)
  line L700 (3.0098, -41.6358) -> (3.0098, -49.2271)
  line L701 (3.0098, -49.2271) -> (1.8574, -49.2271)
  line L702 (1.8574, -49.2271) -> (-2.0338, -43.0828)
  line L703 (-2.0338, -43.0828) -> (-2.0338, -49.2271)
  line L704 (-2.0338, -49.2271) -> (-3.0157, -49.2271)
  line L705 (-3.0157, -49.2271) -> (-3.0157, -41.6358)
  line L706 (14.7693, -41.6358) -> (14.7693, -46.3281)
  spline S518 degree 3 poles (14.7693, -46.3281) (14.7693, -46.8789) (14.8726, -47.3378) (15.0793, -47.7027) knots 0 0 0 0 1 1 1 1
  spline S519 degree 3 poles (15.0793, -47.7027) (15.3863, -48.2535) (15.9031, -48.5295) (16.6296, -48.5295) knots 0 0 0 0 1 1 1 1
  spline S520 degree 3 poles (16.6296, -48.5295) (17.5009, -48.5295) (18.0941, -48.2318) (18.4073, -47.6355) knots 0 0 0 0 1 1 1 1
  spline S521 degree 3 poles (18.4073, -47.6355) (18.5758, -47.312) (18.6605, -46.8758) (18.6605, -46.3281) knots 0 0 0 0 1 1 1 1
  line L707 (18.6605, -46.3281) -> (18.6605, -41.6358)
  line L708 (18.6605, -41.6358) -> (19.7044, -41.6358)
  line L709 (19.7044, -41.6358) -> (19.7044, -45.8992)
  spline S522 degree 3 poles (19.7044, -45.8992) (19.7044, -46.8324) (19.5783, -47.5507) (19.3271, -48.0541) knots 0 0 0 0 1 1 1 1
  spline S523 degree 3 poles (19.3271, -48.0541) (18.8651, -48.9708) (17.9939, -49.4287) (16.7123, -49.4287) knots 0 0 0 0 1 1 1 1
  spline S524 degree 3 poles (16.7123, -49.4287) (15.4307, -49.4287) (14.5605, -48.9708) (14.1026, -48.0541) knots 0 0 0 0 1 1 1 1
  spline S525 degree 3 poles (14.1026, -48.0541) (13.8515, -47.5507) (13.7254, -46.8324) (13.7254, -45.8992) knots 0 0 0 0 1 1 1 1
  line L710 (13.7254, -45.8992) -> (13.7254, -41.6358)
  line L711 (13.7254, -41.6358) -> (14.7693, -41.6358)
  line L712 (17.2032, -39.8375) -> (18.1696, -39.8375)
  line L713 (18.1696, -39.8375) -> (18.1696, -40.9124)
  line L714 (18.1696, -40.9124) -> (17.2032, -40.9124)
  line L715 (17.2032, -40.9124) -> (17.2032, -39.8375)
  line L716 (15.4979, -39.8375) -> (16.4643, -39.8375)
  line L717 (16.4643, -39.8375) -> (16.4643, -40.9124)
  line L718 (16.4643, -40.9124) -> (15.4979, -40.9124)
  line L719 (15.4979, -40.9124) -> (15.4979, -39.8375)
  line L720 (30.3218, -41.6358) -> (31.5362, -41.6358)
  line L721 (31.5362, -41.6358) -> (35.3706, -47.7853)
  line L722 (35.3706, -47.7853) -> (35.3706, -41.6358)
  line L723 (35.3706, -41.6358) -> (36.3473, -41.6358)
  line L724 (36.3473, -41.6358) -> (36.3473, -49.2271)
  line L725 (36.3473, -49.2271) -> (35.1949, -49.2271)
  line L726 (35.1949, -49.2271) -> (31.3037, -43.0828)
  line L727 (31.3037, -43.0828) -> (31.3037, -49.2271)
  line L728 (31.3037, -49.2271) -> (30.3218, -49.2271)
  line L729 (30.3218, -49.2271) -> (30.3218, -41.6358)
  line L730 (49.5754, -41.6358) -> (50.6141, -41.6358)
  line L731 (50.6141, -41.6358) -> (50.6141, -49.2271)
  line L732 (50.6141, -49.2271) -> (49.5754, -49.2271)
  line L733 (49.5754, -49.2271) -> (49.5754, -41.6358)
  line L734 (64.05, -41.6358) -> (69.5845, -41.6358)
  line L735 (69.5845, -41.6358) -> (69.5845, -42.566)
  line L736 (69.5845, -42.566) -> (65.0525, -42.566)
  line L737 (65.0525, -42.566) -> (65.0525, -44.8708)
  line L738 (65.0525, -44.8708) -> (69.2435, -44.8708)
  line L739 (69.2435, -44.8708) -> (69.2435, -45.7493)
  line L740 (69.2435, -45.7493) -> (65.0525, -45.7493)
  line L741 (65.0525, -45.7493) -> (65.0525, -48.3228)
  line L742 (65.0525, -48.3228) -> (69.662, -48.3228)
  line L743 (69.662, -48.3228) -> (69.662, -49.2271)
  line L744 (69.662, -49.2271) -> (64.05, -49.2271)
  line L745 (64.05, -49.2271) -> (64.05, -41.6358)
  line L746 (81.2066, -41.6358) -> (82.2349, -41.6358)
  line L747 (82.2349, -41.6358) -> (82.2349, -48.3228)
  line L748 (82.2349, -48.3228) -> (86.0796, -48.3228)
  line L749 (86.0796, -48.3228) -> (86.0796, -49.2271)
  line L750 (86.0796, -49.2271) -> (81.2066, -49.2271)
  line L751 (81.2066, -49.2271) -> (81.2066, -41.6358)
  line L752 (-86.3336, -66.8746) -> (-81.6776, -61.0403)
  line L753 (-81.6776, -61.0403) -> (-85.9925, -61.0403)
  line L754 (-85.9925, -61.0403) -> (-85.9925, -60.136)
  line L755 (-85.9925, -60.136) -> (-80.3546, -60.136)
  line L756 (-80.3546, -60.136) -> (-80.3546, -61.0197)
  line L757 (-80.3546, -61.0197) -> (-85.0365, -66.8229)
  line L758 (-85.0365, -66.8229) -> (-80.3546, -66.8229)
  line L759 (-80.3546, -66.8229) -> (-80.3546, -67.7273)
  line L760 (-80.3546, -67.7273) -> (-86.3336, -67.7273)
  line L761 (-86.3336, -67.7273) -> (-86.3336, -66.8746)
  line L762 (-65.5018, -64.6164) -> (-66.6542, -61.2626)
  line L763 (-66.6542, -61.2626) -> (-67.8789, -64.6164)
  line L764 (-67.8789, -64.6164) -> (-65.5018, -64.6164)
  line L765 (-67.1916, -60.136) -> (-66.0289, -60.136)
  line L766 (-66.0289, -60.136) -> (-63.2745, -67.7273)
  line L767 (-63.2745, -67.7273) -> (-64.4011, -67.7273)
  line L768 (-64.4011, -67.7273) -> (-65.1711, -65.4535)
  line L769 (-65.1711, -65.4535) -> (-68.1735, -65.4535)
  line L770 (-68.1735, -65.4535) -> (-68.9951, -67.7273)
  line L771 (-68.9951, -67.7273) -> (-70.0493, -67.7273)
  line L772 (-70.0493, -67.7273) -> (-67.1916, -60.136)
  line L773 (-66.2924, -58.3377) -> (-65.3261, -58.3377)
  line L774 (-65.3261, -58.3377) -> (-65.3261, -59.4125)
  line L775 (-65.3261, -59.4125) -> (-66.2924, -59.4125)
  line L776 (-66.2924, -59.4125) -> (-66.2924, -58.3377)
  line L777 (-67.9978, -58.3377) -> (-67.0314, -58.3377)
  line L778 (-67.0314, -58.3377) -> (-67.0314, -59.4125)
  line L779 (-67.0314, -59.4125) -> (-67.9978, -59.4125)
  line L780 (-67.9978, -59.4125) -> (-67.9978, -58.3377)
  line L781 (-53.0219, -60.136) -> (-51.8075, -60.136)
  line L782 (-51.8075, -60.136) -> (-47.9732, -66.2855)
  line L783 (-47.9732, -66.2855) -> (-47.9732, -60.136)
  line L784 (-47.9732, -60.136) -> (-46.9965, -60.136)
  line L785 (-46.9965, -60.136) -> (-46.9965, -67.7273)
  line L786 (-46.9965, -67.7273) -> (-48.1489, -67.7273)
  line L787 (-48.1489, -67.7273) -> (-52.0401, -61.583)
  line L788 (-52.0401, -61.583) -> (-52.0401, -67.7273)
  line L789 (-52.0401, -67.7273) -> (-53.0219, -67.7273)
  line L790 (-53.0219, -67.7273) -> (-53.0219, -60.136)
  line L791 (-33.7683, -60.136) -> (-32.7296, -60.136)
  line L792 (-32.7296, -60.136) -> (-32.7296, -67.7273)
  line L793 (-32.7296, -67.7273) -> (-33.7683, -67.7273)
  line L794 (-33.7683, -67.7273) -> (-33.7683, -60.136)
  line L795 (-19.2938, -60.136) -> (-13.7592, -60.136)
  line L796 (-13.7592, -60.136) -> (-13.7592, -61.0662)
  line L797 (-13.7592, -61.0662) -> (-18.2912, -61.0662)
  line L798 (-18.2912, -61.0662) -> (-18.2912, -63.371)
  line L799 (-18.2912, -63.371) -> (-14.1003, -63.371)
  line L800 (-14.1003, -63.371) -> (-14.1003, -64.2495)
  line L801 (-14.1003, -64.2495) -> (-18.2912, -64.2495)
  line L802 (-18.2912, -64.2495) -> (-18.2912, -66.8229)
  line L803 (-18.2912, -66.8229) -> (-13.6817, -66.8229)
  line L804 (-13.6817, -66.8229) -> (-13.6817, -67.7273)
  line L805 (-13.6817, -67.7273) -> (-19.2938, -67.7273)
  line L806 (-19.2938, -67.7273) -> (-19.2938, -60.136)
  spline S526 degree 3 poles (0.1831, -59.9293) (1.1443, -59.9293) (1.8905, -60.1825) (2.4207, -60.6889) knots 0 0 0 0 1 1 1 1
  spline S527 degree 3 poles (2.4207, -60.6889) (2.9509, -61.1954) (3.2454, -61.7711) (3.3043, -62.4149) knots 0 0 0 0 1 1 1 1
  line L807 (3.3043, -62.4149) -> (2.3018, -62.4149)
  spline S528 degree 3 poles (2.3018, -62.4149) (2.1881, -61.9261) (1.9618, -61.5385) (1.6228, -61.2522) knots 0 0 0 0 1 1 1 1
  spline S529 degree 3 poles (1.6228, -61.2522) (1.2828, -60.9659) (0.8063, -60.8233) (0.1934, -60.8233) knots 0 0 0 0 1 1 1 1
  spline S530 degree 3 poles (0.1934, -60.8233) (-0.5538, -60.8233) (-1.1574, -61.0858) (-1.6184, -61.6109) knots 0 0 0 0 1 1 1 1
  spline S531 degree 3 poles (-1.6184, -61.6109) (-2.0783, -62.1369) (-2.3077, -62.942) (-2.3077, -64.0272) knots 0 0 0 0 1 1 1 1
  spline S532 degree 3 poles (-2.3077, -64.0272) (-2.3077, -64.9161) (-2.1, -65.6375) (-1.6845, -66.1894) knots 0 0 0 0 1 1 1 1
  spline S533 degree 3 poles (-1.6845, -66.1894) (-1.2701, -66.7423) (-0.651, -67.0193) (0.1727, -67.0193) knots 0 0 0 0 1 1 1 1
  spline S534 degree 3 poles (0.1727, -67.0193) (0.9303, -67.0193) (1.5081, -66.7279) (1.9039, -66.146) knots 0 0 0 0 1 1 1 1
  spline S535 degree 3 poles (1.9039, -66.146) (2.1137, -65.839) (2.2708, -65.4359) (2.3742, -64.9368) knots 0 0 0 0 1 1 1 1
  line L808 (2.3742, -64.9368) -> (3.3767, -64.9368)
  spline S536 degree 3 poles (3.3767, -64.9368) (3.2868, -65.7357) (2.9912, -66.4064) (2.4878, -66.947) knots 0 0 0 0 1 1 1 1
  spline S537 degree 3 poles (2.4878, -66.947) (1.8853, -67.5981) (1.0719, -67.9236) (0.0487, -67.9236) knots 0 0 0 0 1 1 1 1
  spline S538 degree 3 poles (0.0487, -67.9236) (-0.8329, -67.9236) (-1.5739, -67.657) (-2.1734, -67.1227) knots 0 0 0 0 1 1 1 1
  spline S539 degree 3 poles (-2.1734, -67.1227) (-2.9619, -66.4168) (-3.3568, -65.3264) (-3.3568, -63.8515) knots 0 0 0 0 1 1 1 1
  spline S540 degree 3 poles (-3.3568, -63.8515) (-3.3568, -62.7322) (-3.0601, -61.8134) (-2.4679, -61.0972) knots 0 0 0 0 1 1 1 1
  spline S541 degree 3 poles (-2.4679, -61.0972) (-1.8271, -60.3189) (-0.9435, -59.9293) (0.1831, -59.9293) knots 0 0 0 0 1 1 1 1
  line L809 (13.6789, -60.136) -> (14.7176, -60.136)
  line L810 (14.7176, -60.136) -> (14.7176, -63.2728)
  line L811 (14.7176, -63.2728) -> (18.6657, -63.2728)
  line L812 (18.6657, -63.2728) -> (18.6657, -60.136)
  line L813 (18.6657, -60.136) -> (19.7044, -60.136)
  line L814 (19.7044, -60.136) -> (19.7044, -67.7273)
  line L815 (19.7044, -67.7273) -> (18.6657, -67.7273)
  line L816 (18.6657, -67.7273) -> (18.6657, -64.1771)
  line L817 (18.6657, -64.1771) -> (14.7176, -64.1771)
  line L818 (14.7176, -64.1771) -> (14.7176, -67.7273)
  line L819 (14.7176, -67.7273) -> (13.6789, -67.7273)
  line L820 (13.6789, -67.7273) -> (13.6789, -60.136)
  line L821 (30.7125, -60.136) -> (36.247, -60.136)
  line L822 (36.247, -60.136) -> (36.247, -61.0662)
  line L823 (36.247, -61.0662) -> (31.715, -61.0662)
  line L824 (31.715, -61.0662) -> (31.715, -63.371)
  line L825 (31.715, -63.371) -> (35.906, -63.371)
  line L826 (35.906, -63.371) -> (35.906, -64.2495)
  line L827 (35.906, -64.2495) -> (31.715, -64.2495)
  line L828 (31.715, -64.2495) -> (31.715, -66.8229)
  line L829 (31.715, -66.8229) -> (36.3245, -66.8229)
  line L830 (36.3245, -66.8229) -> (36.3245, -67.7273)
  line L831 (36.3245, -67.7273) -> (30.7125, -67.7273)
  line L832 (30.7125, -67.7273) -> (30.7125, -60.136)
  line L833 (48.1068, -60.136) -> (48.1068, -64.8282)
  spline S542 degree 3 poles (48.1068, -64.8282) (48.1068, -65.3791) (48.2101, -65.838) (48.4168, -66.2028) knots 0 0 0 0 1 1 1 1
  spline S543 degree 3 poles (48.4168, -66.2028) (48.7238, -66.7537) (49.2406, -67.0296) (49.9671, -67.0296) knots 0 0 0 0 1 1 1 1
  spline S544 degree 3 poles (49.9671, -67.0296) (50.8384, -67.0296) (51.4316, -66.732) (51.7448, -66.1356) knots 0 0 0 0 1 1 1 1
  spline S545 degree 3 poles (51.7448, -66.1356) (51.9133, -65.8122) (51.998, -65.376) (51.998, -64.8282) knots 0 0 0 0 1 1 1 1
  line L834 (51.998, -64.8282) -> (51.998, -60.136)
  line L835 (51.998, -60.136) -> (53.0419, -60.136)
  line L836 (53.0419, -60.136) -> (53.0419, -64.3993)
  spline S546 degree 3 poles (53.0419, -64.3993) (53.0419, -65.3326) (52.9158, -66.0509) (52.6646, -66.5542) knots 0 0 0 0 1 1 1 1
  spline S547 degree 3 poles (52.6646, -66.5542) (52.2026, -67.471) (51.3314, -67.9288) (50.0498, -67.9288) knots 0 0 0 0 1 1 1 1
  spline S548 degree 3 poles (50.0498, -67.9288) (48.7682, -67.9288) (47.898, -67.471) (47.4401, -66.5542) knots 0 0 0 0 1 1 1 1
  spline S549 degree 3 poles (47.4401, -66.5542) (47.189, -66.0509) (47.0629, -65.3326) (47.0629, -64.3993) knots 0 0 0 0 1 1 1 1
  line L837 (47.0629, -64.3993) -> (47.0629, -60.136)
  line L838 (47.0629, -60.136) -> (48.1068, -60.136)
  line L839 (64.3466, -60.136) -> (69.6124, -60.136)
  line L840 (69.6124, -60.136) -> (69.6124, -61.0662)
  line L841 (69.6124, -61.0662) -> (65.375, -61.0662)
  line L842 (65.375, -61.0662) -> (65.375, -63.371)
  line L843 (65.375, -63.371) -> (69.1008, -63.371)
  line L844 (69.1008, -63.371) -> (69.1008, -64.2753)
  line L845 (69.1008, -64.2753) -> (65.375, -64.2753)
  line L846 (65.375, -64.2753) -> (65.375, -67.7273)
  line L847 (65.375, -67.7273) -> (64.3466, -67.7273)
  line L848 (64.3466, -67.7273) -> (64.3466, -60.136)
  line L849 (82.9129, -60.136) -> (83.9516, -60.136)
  line L850 (83.9516, -60.136) -> (83.9516, -67.7273)
  line L851 (83.9516, -67.7273) -> (82.9129, -67.7273)
  line L852 (82.9129, -67.7273) -> (82.9129, -60.136)
  line L853 (-86.3336, -85.3748) -> (-81.6776, -79.5405)
  line L854 (-81.6776, -79.5405) -> (-85.9925, -79.5405)
  line L855 (-85.9925, -79.5405) -> (-85.9925, -78.6362)
  line L856 (-85.9925, -78.6362) -> (-80.3546, -78.6362)
  line L857 (-80.3546, -78.6362) -> (-80.3546, -79.5198)
  line L858 (-80.3546, -79.5198) -> (-85.0365, -85.3231)
  line L859 (-85.0365, -85.3231) -> (-80.3546, -85.3231)
  line L860 (-80.3546, -85.3231) -> (-80.3546, -86.2274)
  line L861 (-80.3546, -86.2274) -> (-86.3336, -86.2274)
  line L862 (-86.3336, -86.2274) -> (-86.3336, -85.3748)
  line L863 (-70.3615, -78.6362) -> (-68.93, -84.8115)
  line L864 (-68.93, -84.8115) -> (-67.2144, -78.6362)
  line L865 (-67.2144, -78.6362) -> (-66.0981, -78.6362)
  line L866 (-66.0981, -78.6362) -> (-64.3825, -84.8115)
  line L867 (-64.3825, -84.8115) -> (-62.951, -78.6362)
  line L868 (-62.951, -78.6362) -> (-61.8245, -78.6362)
  line L869 (-61.8245, -78.6362) -> (-63.8192, -86.2274)
  line L870 (-63.8192, -86.2274) -> (-64.8993, -86.2274)
  line L871 (-64.8993, -86.2274) -> (-66.6511, -79.9333)
  line L872 (-66.6511, -79.9333) -> (-68.4132, -86.2274)
  line L873 (-68.4132, -86.2274) -> (-69.4933, -86.2274)
  line L874 (-69.4933, -86.2274) -> (-71.4777, -78.6362)
  line L875 (-71.4777, -78.6362) -> (-70.3615, -78.6362)
  spline S550 degree 3 poles (-50.0392, -78.4295) (-48.6987, -78.4295) (-47.7065, -78.8604) (-47.0626, -79.7214) knots 0 0 0 0 1 1 1 1
  spline S551 degree 3 poles (-47.0626, -79.7214) (-46.5593, -80.3932) (-46.3081, -81.2531) (-46.3081, -82.3) knots 0 0 0 0 1 1 1 1
  spline S552 degree 3 poles (-46.3081, -82.3) (-46.3081, -83.4338) (-46.5955, -84.3754) (-47.1711, -85.1267) knots 0 0 0 0 1 1 1 1